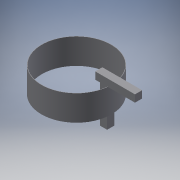
# Autodesk Inventor part: Burner-Placeholder
Saved by Autodesk Inventor 2017 (Build 210142000, 142)
## iProperties
Created: 2017-08-30
Part Number: Burner-Placeholder
Material: Generic
Document SubType Name: Modeling
Designer: Trent
Density: 1 g/cm^3
Appearance: Default
Author: Trent
Autodesk Inventor part; units mm, degrees
ref_plane "YZ Plane" through (0, 0, 0) normal (1, 0, 0) x (0, 1, 0)
ref_plane "XZ Plane" through (0, 0, 0) normal (0, 1, 0) x (-1, 0, 0)
ref_plane "XY Plane" through (0, 0, 0) normal (0, 0, 1) x (1, 0, 0)
sketch "Sketch1" plane through (0, 0, 0) normal (0, 1, 0) x (-1, 0, 0)
  circle A0 centre (0, 0) radius 139.7
  circle A1 centre (0, 0) radius 138.1125
  dimension "d0" = 279.4
  dimension "d1" = 276.225
  constraints: 2 centre point, 2 coincident
  measures "d0" diameter of A0
  measures "d1" diameter of A1
extrude "Extrusion1" add sketch "Sketch1" along normal blind 101.6
sketch "Sketch2" plane through (0, 101.6, 0) normal (0, 1, 0) x (1, 0, 0)
  line L0 (88.9, 14.2875) -> (247.65, 14.2875)
  line L1 (247.65, 14.2875) -> (247.65, -14.2875)
  line L2 (247.65, -14.2875) -> (88.9, -14.2875)
  line L3 (88.9, -14.2875) -> (88.9, 14.2875)
  line L4 (88.9, 14.2875) -> (247.65, -14.2875) construction
  line L5 (247.65, 14.2875) -> (88.9, -14.2875) construction
  circle A0 centre (0, 0) radius 139.7 projected
  point P0 (168.275, 0)
  point P1 (168.275, 0)
  point P2 (139.7, 0)
  dimension "d4" = 158.75
  dimension "d5" = 28.575
  dimension "d7" = 107.95
  constraints: 12 end point, 3 horizontal alignment, 3 midpoint, 2 parallel, 1 horizontal, 1 perpendicular, 1 other
  measures "d4" distance of L1.end L2.end
  measures "d5" distance of L0.end L1.end
  measures "d7" distance from line of L1 point (139.7, 0)
extrude "Extrusion2" add sketch "Sketch2" along normal blind 28.575 contours L0 A0 L2 L3 | L0 L1 L2 A0 picked at (105.8333, 0)
sketch "Sketch3" plane through (0, 101.6, 0) normal (0, -1, 0) x (1, 0, 0)
  line L0 (247.65, -14.2875) -> (88.9, -14.2875) projected
  line L1 (107.95, 14.2875) -> (136.525, 14.2875)
  line L2 (136.525, 14.2875) -> (136.525, -14.2875)
  line L3 (136.525, -14.2875) -> (107.95, -14.2875)
  line L4 (107.95, -14.2875) -> (107.95, 14.2875)
  line L5 (107.95, 14.2875) -> (136.525, -14.2875) construction
  line L6 (136.525, 14.2875) -> (107.95, -14.2875) construction
  line L7 (88.9, 14.2875) -> (88.9, -14.2875) projected
  line L8 (137.3715, 14.2875) -> (88.9, 14.2875) projected
  point P0 (0, 0)
  point P1 (122.2375, 0)
  dimension "d10" = 28.575
  dimension "d11" = 19.05
  constraints: 12 end point, 2 midpoint, 2 parallel, 1 collinear, 1 horizontal, 1 perpendicular, 1 point on line
  measures "d10" distance of L2.end L3.end
  measures "d11" distance between parallel lines of L7 L4
extrude "Extrusion3" add sketch "Sketch3" along normal blind 149.225 contours L0 L4 L1 L2
pattern_circular "Circular Pattern1" count 3 over 360 about axis through (0, 0, 0) along (0, 1, 0) of "Extrusion2", "Extrusion3"
body "Solid1"
